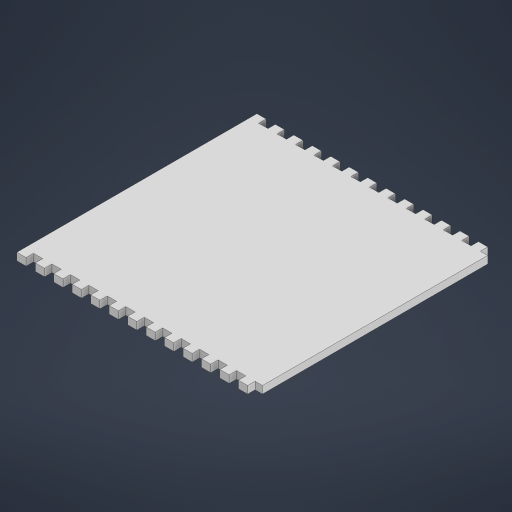
# Autodesk Inventor part: Top cover with groves
Saved by Autodesk Inventor 2023 (Build 270158030, 158C)
## iProperties
Created: 2022-06-21
Part Number: Top cover with groves
Material: Generic
Document SubType Name: Modeling
Designer: Simon
Density: 1 g/cm^3
Appearance: Default
Author: Simon
Autodesk Inventor part; units mm, degrees
ref_plane "YZ Plane" through (0, 0, 0) normal (1, 0, 0) x (0, 1, 0)
ref_plane "XZ Plane" through (0, 0, 0) normal (0, 1, 0) x (-1, 0, 0)
ref_plane "XY Plane" through (0, 0, 0) normal (0, 0, 1) x (1, 0, 0)
sketch "Sketch1" plane through (0, 0, 0) normal (0, 1, 0) x (-1, 0, 0)
  line L0 (-19, 126) -> (-19, 4)
  line L1 (-15, 126) -> (-19, 126)
  line L2 (-15, 126) -> (-15, 130)
  line L3 (-10, 130) -> (-15, 130)
  line L4 (-10, 126) -> (-10, 130)
  line L5 (-5, 126) -> (-10, 126)
  line L6 (-5, 126) -> (-5, 130)
  line L7 (0, 130) -> (-5, 130)
  line L8 (0, 126) -> (0, 130)
  line L9 (5, 126) -> (0, 126)
  line L10 (5, 126) -> (5, 130)
  line L11 (10, 130) -> (5, 130)
  line L12 (10, 126) -> (10, 130)
  line L13 (15, 126) -> (10, 126)
  line L14 (15, 126) -> (15, 130)
  line L15 (20, 130) -> (15, 130)
  line L16 (20, 126) -> (20, 130)
  line L17 (25, 126) -> (20, 126)
  line L18 (25, 126) -> (25, 130)
  line L19 (30, 130) -> (25, 130)
  line L20 (30, 126) -> (30, 130)
  line L21 (35, 126) -> (30, 126)
  line L22 (35, 126) -> (35, 130)
  line L23 (40, 130) -> (35, 130)
  line L24 (40, 126) -> (40, 130)
  line L25 (45, 126) -> (40, 126)
  line L26 (45, 126) -> (45, 130)
  line L27 (50, 130) -> (45, 130)
  line L28 (50, 126) -> (50, 130)
  line L29 (55, 126) -> (50, 126)
  line L30 (55, 126) -> (55, 130)
  line L31 (60, 130) -> (55, 130)
  line L32 (60, 126) -> (60, 130)
  line L33 (65, 126) -> (60, 126)
  line L34 (65, 126) -> (65, 130)
  line L35 (70, 130) -> (65, 130)
  line L36 (70, 126) -> (70, 130)
  line L37 (75, 126) -> (70, 126)
  line L38 (75, 126) -> (75, 130)
  line L39 (80, 130) -> (75, 130)
  line L40 (80, 126) -> (80, 130)
  line L41 (85, 126) -> (80, 126)
  line L42 (85, 126) -> (85, 130)
  line L43 (90, 130) -> (85, 130)
  line L44 (90, 126) -> (90, 130)
  line L45 (95, 126) -> (90, 126)
  line L46 (95, 126) -> (95, 130)
  line L47 (100, 130) -> (95, 130)
  line L48 (100, 126) -> (100, 130)
  line L49 (105, 126) -> (100, 126)
  line L50 (105, 126) -> (105, 130)
  line L51 (110, 130) -> (105, 130)
  line L52 (110, 126) -> (110, 130)
  line L53 (110, 65) -> (110, 126)
  line L54 (110, 65) -> (-15, 65)
  line L55 (110, 65) -> (235, 65) construction
  line L56 (-15, 65) -> (-19, 65)
  point P0 (0, 0)
  dimension "d0" = 180
  constraints: 114 end point, 1 collinear, 1 horizontal, 1 midpoint, 1 vertical
  measures "d0" angle of L54 L55
extrude "Extrusion1" add sketch "Sketch1" along normal blind 4
mirror "Mirror1" about plane through (19, 0, 65) normal (0, 0, -1) of "Extrusion1"
body "Solid1"
